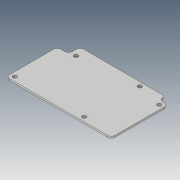
# Autodesk Inventor part: escPlate
Saved by Autodesk Inventor 2018 (Build 220112000, 112)
## iProperties
Created: 2020-02-05
Part Number: escPlate
Material: Generic
Document SubType Name: Modeling
Designer: anirudh.bali
Density: 1 g/cm^3
Appearance: Default
Author: anirudh.bali
Autodesk Inventor part; units mm, degrees
ref_plane "YZ Plane" through (0, 0, 0) normal (1, 0, 0) x (0, 1, 0)
ref_plane "XZ Plane" through (0, 0, 0) normal (0, 1, 0) x (-1, 0, 0)
ref_plane "XY Plane" through (0, 0, 0) normal (0, 0, 1) x (1, 0, 0)
sketch "Sketch1" plane through (0, 0, 0) normal (0, 1, 0) x (-1, 0, 0)
  line L0 (-93.98, 0) -> (-93.98, -44.45)
  line L1 (0, -44.45) -> (0, 0)
  circle A0 centre (-15.24, -46.04) radius 1.75
  circle A1 centre (-67.3, -50.86) radius 1.75
  circle A2 centre (-66.05, -2.54) radius 1.75
  line L2 (0, -44.45) -> (-10.16, -44.45)
  line L3 (-93.98, -44.45) -> (-93.98, -54.61)
  line L4 (-93.98, -54.61) -> (-10.16, -54.61)
  line L5 (-10.16, -54.61) -> (-10.16, -44.45)
  line L6 (-66.05, 1.2192) -> (-93.98, 1.2192)
  line L7 (-93.98, 1.2192) -> (-93.98, 0)
  line L8 (-66.05, 1.2192) -> (0, 1.2192)
  line L9 (0, 1.2192) -> (0, 0)
  line L10 (0, 1.2192) -> (0, -6.5338)
  circle A3 centre (-3.8735, -2.6573) radius 1.75
  line L11 (-93.98, -49.2808) -> (-93.98, -41.5338)
  circle A4 centre (-90.1065, -45.4073) radius 1.75
  constraints: 24 end point, 5 centre point, 2 coincident, 2 collinear, 2 perpendicular, 2 point on line, 1 horizontal, 1 parallel, 1 vertical
extrude "Extrusion1" add sketch "Sketch1" along normal blind 1.5875
fillet "Fillet1" radius 3.175 6 edges at (0, 0.7937, 1.2192) (0, 0.7937, -44.45) (10.16, 0.7937, -44.45) (10.16, 0.7937, -54.61) (93.98, 0.7937, 1.2192) (93.98, 0.7937, -54.61)
sketch "Sketch2" plane through (0, 1.5875, 0) normal (0, 1, 0) x (1, 0, 0)
  circle A0 centre (90.1065, 45.4073) radius 1.75 projected
  arc A1 (93.98, 45.4073) -> (90.1065, 49.2808) centre (90.1065, 45.4073) ccw
  line L0 (93.98, 1.9558) -> (93.98, 51.435) projected
  line L1 (86.233, 49.2808) -> (86.233, 54.61)
  line L2 (90.805, 54.61) -> (13.335, 54.61) projected
  line L3 (90.1065, 49.2808) -> (86.233, 49.2808)
  arc A2 (93.98, 51.435) -> (90.805, 54.61) centre (90.805, 51.435) ccw projected
  arc A3 (93.98, 51.435) -> (90.805, 54.61) centre (90.805, 51.435) ccw
  line L4 (93.98, 45.4073) -> (93.98, 51.435)
  line L5 (90.805, 54.61) -> (86.233, 54.61)
  point P0 (0, 0)
  constraints: 8 end point, 5 point on circle, 5 tangent, 4 point on line, 2 centre point, 2 coincident, 2 vertical, 1 collinear, 1 perpendicular
extrude "Extrusion2" cut sketch "Sketch2" against normal blind 25.4 contours A1 L3 L1 L2 A2 L0
fillet "Fillet2" radius 3.175 2 edges at (86.233, 0.7937, -49.2808) (86.233, 0.7937, -54.61)
body "Solid1"
